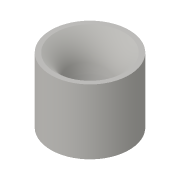
# Autodesk Inventor part: nozzle 8in version 1
Saved by Autodesk Inventor 2016 SP1 (Build 200210100, 210)
## iProperties
Created: 2016-06-14
Part Number: nozzle 8in version 1
Material: Generic
Document SubType Name: Modeling
Designer: Neal
Density: 1 g/cm^3
Appearance: Default
Author: Neal
Autodesk Inventor part; units mm, degrees
ref_plane "YZ Plane" through (0, 0, 0) normal (1, 0, 0) x (0, 1, 0)
ref_plane "XZ Plane" through (0, 0, 0) normal (0, 1, 0) x (-1, 0, 0)
ref_plane "XY Plane" through (0, 0, 0) normal (0, 0, 1) x (1, 0, 0)
sketch "Sketch1" plane through (0, 0, 0) normal (0, 0, 1) x (1, 0, 0)
  line L0 (-68.3895, -51.5874) -> (-9.652, -51.5874) construction
  line L1 (-54.61, 44.1185) -> (-48.3044, 44.1185)
  line L2 (-54.61, 44.1185) -> (-9.6509, 44.1185) construction
  line L3 (-54.61, 44.1185) -> (36.0172, 44.1185) construction
  line L4 (-75.5396, 46.8376) -> (-27.9582, 46.8376) construction
  line L5 (-75.5396, 46.8376) -> (-24.3567, 46.8376) construction
  line L6 (-75.5396, 46.8376) -> (-39.9094, 46.8376) construction
  line L7 (-85.2325, 14.4461) -> (-72.647, 14.4461)
  line L8 (-85.2325, 14.4461) -> (-78.8825, 14.4461)
  line L9 (-47.0755, -46.5087) -> (-40.7255, -46.5087)
  line L10 (-54.61, -46.5087) -> (-47.0755, -46.5087)
  arc A0 (-29.1336, -3.2472) -> (-28.7009, 0.0398) centre (-41.4009, 0.0398) ccw
  line L11 (-72.647, 14.4461) -> (-72.647, -49.0501)
  line L12 (-85.2325, 7.0204) -> (-85.2325, -49.0501)
  line L13 (-78.8825, 7.0204) -> (-85.2325, 7.0204)
  line L14 (-78.8825, 14.4461) -> (-78.8825, 7.0204)
  line L15 (-54.61, 44.1185) -> (-54.61, -46.5087)
  line L16 (-29.1336, -3.2472) -> (-78.2122, -186.4111)
  line L17 (-78.997, -110.2264) -> (-72.647, -110.2264)
  line L18 (-72.647, -141.9758) -> (-66.3058, -141.9758)
  line L19 (-78.997, -110.2264) -> (-78.997, -186.4111)
  line L20 (-72.647, -49.0501) -> (-85.2325, -49.0501)
  line L21 (-72.6469, -48.8475) -> (-59.9469, -48.8475) construction
  line L22 (-85.2325, 26.3534) -> (-71.1236, 26.3534)
  line L23 (-71.1236, 26.3534) -> (-64.7736, 26.3534)
  line L24 (-64.7736, 26.3534) -> (-64.7736, -49.0592)
  line L25 (-64.7736, -49.0592) -> (-64.7736, -112.5592)
  line L26 (-64.7736, -112.5592) -> (-58.4236, -112.5592)
  line L27 (-85.2325, 26.3534) -> (-85.2325, 42.2284)
  line L28 (-85.2325, 42.2284) -> (-78.2952, 42.2284)
  line L29 (-78.2952, 42.2284) -> (-78.2952, 58.1034)
  line L30 (-78.2952, 58.1034) -> (-48.3044, 44.1185)
  line L31 (-77.6767, 58.2932) -> (49.3233, 58.2932) construction
  arc A1 (-28.7009, 0.0398) -> (-48.3044, 44.1185) centre (-75.5766, 5.5909) ccw
  line L32 (-78.997, -186.4111) -> (-78.2122, -186.4111)
  line L33 (-72.6558, -49.0501) -> (-72.647, -49.0501)
  line L34 (-85.2325, 26.3534) -> (-85.2325, 14.4461)
  line L35 (-72.647, -49.0501) -> (-72.647, -110.2264)
  line L36 (-72.647, -110.2264) -> (-72.647, -141.9758)
  line L37 (0, -235.352) -> (0, 107.2341) projected
  point P0 (0, 0)
  point P1 (-9.6509, 0.0398)
  dimension "d5" = 12.7
  dimension "d7" = 6.35
  dimension "d8" = 105
  dimension "d23" = 76.1847
  dimension "d26" = 31.7495
  dimension "d30" = 90
  dimension "d33" = 6.35
  dimension "d51" = 6.35
  dimension "d54" = 6.35
  dimension "d55" = 15.875
  dimension "d56" = 6.9374
  dimension "d57" = 15.875
  dimension "d60" = 25
  dimension "d62" = 28.7008
  dimension "d63" = 54.61
  dimension "d64" = 6.3056
  constraints: 75 end point, 16 horizontal, 8 perpendicular, 8 vertical, 6 point on line, 4 point on circle, 2 centre point, 2 horizontal alignment, 1 tangent
  measures "d5" radius of A0
  measures "d7" distance of L10.end L9.end
  measures "d8" angle of L9 L16
  measures "d23" distance of L19.end L17.start
  measures "d26" distance between parallel lines of L17 L18
  measures "d30" angle of L15 L3
  measures "d33" distance of L17.end L17.start
  measures "d51" distance of L22.end L23.end
  measures "d54" distance of L25.end L26.end
  measures "d55" distance of L22.start L27.end
  measures "d56" distance of L27.end L28.end
  measures "d57" distance of L28.end L29.end
  measures "d60" angle of L30 L31
  measures "d62" distance of point (0, 0) A0.end
  measures "d63" horizontal distance of point (0, 0) L15.start
  measures "d64" distance of L1.end L15.start
revolve "Revolution1" add sketch "Sketch1" angle 360 about axis through (0, -10, 0) along (0, 1, 0) contours L1 A1 A0 L16 L9 L10 L15
body "Solid1"
